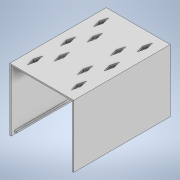
# Autodesk Inventor part: netzteil_halter_oben
Saved by Autodesk Inventor 2021 (Build 250183000, 183)
## iProperties
Created: 2021-11-10
Part Number: netzteil_halter_oben
Material: Generisch
Document SubType Name: Modeling
Designer: Simon
Density: 1 g/cm^3
Appearance: Vorgabe
Author: Simon
Autodesk Inventor part; units mm, degrees
ref_plane "YZ Plane" through (0, 0, 0) normal (1, 0, 0) x (0, 1, 0)
ref_plane "XZ Plane" through (0, 0, 0) normal (0, 1, 0) x (-1, 0, 0)
ref_plane "XY Plane" through (0, 0, 0) normal (0, 0, 1) x (1, 0, 0)
sketch "Skizze1" plane through (0, 0, 0) normal (0, 0, 1) x (1, 0, 0)
  line L0 (-63, 61.5) -> (63, 61.5)
  line L1 (63, 61.5) -> (63, -61.5)
  line L2 (63, -61.5) -> (-63, -61.5)
  line L3 (-63, -61.5) -> (-63, 61.5)
  point P0 (0, 0)
  point P1 (0, 61.5)
  point P2 (-63, 0)
  dimension "d0" = 123
  dimension "d1" = 126
  constraints: 8 end point, 2 midpoint, 2 parallel, 1 horizontal, 1 horizontal alignment, 1 perpendicular, 1 vertical alignment
  measures "d0" distance of L0.end L1.end
  measures "d1" distance between parallel lines of L1 L3
extrude "Extrusion1" add sketch "Skizze1" along normal blind 5
sketch "Skizze3" plane through (0, 0, 5) normal (0, 0, 1) x (1, 0, 0)
  line L0 (5, -51.5) -> (5, 58.5) construction
  line L1 (5, 58.5) -> (10.5, 58.5) construction
  line L2 (10.5, 58.5) -> (10.5, -51.5) construction
  line L3 (10.5, -51.5) -> (60, -51.5) construction
  line L4 (60, -51.5) -> (60, -54.5) construction
  line L5 (60, -54.5) -> (56, -54.5) construction
  line L6 (56, -54.5) -> (56, -58.5) construction
  line L7 (56, -58.5) -> (60, -58.5) construction
  line L8 (60, -58.5) -> (60, -61.5) construction
  line L9 (60, -61.5) -> (-60, -61.5) construction
  line L10 (-60, -61.5) -> (-60, -58.5) construction
  line L11 (-60, -58.5) -> (-56, -58.5) construction
  line L12 (-56, -58.5) -> (-56, -54.5) construction
  line L13 (-56, -54.5) -> (-60, -54.5) construction
  line L14 (-60, -54.5) -> (-60, -51.5) construction
  line L15 (-60, -51.5) -> (5, -51.5) construction
  line L16 (-63, -61.5) -> (63, -61.5) projected
  line L17 (63, -61.5) -> (63, 61.5) projected
  line L18 (-63, -61.5) -> (-60.5, -61.5)
  line L19 (-60.5, -58) -> (-60.5, -61.5)
  line L20 (-60.5, -58) -> (-56.5, -58)
  line L21 (-56.5, -58) -> (-56.5, -55)
  line L22 (-56.5, -55) -> (-60.5, -55)
  line L23 (-60.5, -55) -> (-60.5, 56.5)
  line L24 (60.5, 56.5) -> (60.5, -55)
  line L25 (60.5, -55) -> (56.5, -55)
  line L26 (56.5, -55) -> (56.5, -58)
  line L27 (56.5, -58) -> (60.5, -58)
  line L28 (60.5, -61.5) -> (60.5, -58)
  line L29 (60.5, -61.5) -> (63, -61.5)
  line L30 (63, -61.5) -> (63, 61.5)
  line L31 (63, 61.5) -> (-63, 61.5) projected
  line L32 (63, 61.5) -> (-63, 61.5)
  line L33 (-63, 61.5) -> (-63, -61.5)
  line L34 (4, 56.5) -> (4, 59)
  line L35 (4, 59) -> (11.5, 59)
  line L36 (11.5, 59) -> (11.5, 56.5)
  line L37 (-60.5, 56.5) -> (4, 56.5)
  line L38 (11.5, 56.5) -> (60.5, 56.5)
  point P0 (0, 0)
  dimension "d4" = 4
  dimension "d5" = 4
  dimension "d6" = 3
  dimension "d7" = 10
  dimension "d8" = 120
  dimension "d10" = 5.5
  dimension "d11" = 120
  dimension "d13" = 0.5
  dimension "d14" = 0.5
  dimension "d15" = 0.5
  dimension "d16" = 0.5
  dimension "d17" = 0.5
  dimension "d18" = 0.5
  dimension "d19" = 0.5
  dimension "d20" = 1
  dimension "d21" = 1
  dimension "d22" = 5
  dimension "d25" = 65
  constraints: 72 end point, 30 perpendicular, 15 point on line, 4 equal length, 2 collinear, 2 horizontal, 1 vertical
  measures "d4" distance of L10.end L11.end
  measures "d5" distance of L11.end L12.end
  measures "d6" distance between parallel lines of L9 L11
  measures "d7" distance between parallel lines of L15 L9
  measures "d8" distance of L8.end L9.end
  measures "d10" distance between parallel lines of L0 L2
  measures "d11" distance between parallel lines of L1 L9
  measures "d13" distance between parallel lines of L10 L19
  measures "d14" distance between parallel lines of L20 L11
  measures "d15" distance between parallel lines of L12 L21
  measures "d16" distance between parallel lines of L13 L22
  measures "d17" distance between parallel lines of L6 L26
  measures "d18" distance between parallel lines of L8 L28
  measures "d19" distance between parallel lines of L1 L35
  measures "d20" distance between parallel lines of L34 L0
  measures "d21" distance between parallel lines of L2 L36
  measures "d22" distance between parallel lines of L32 L38
  measures "d25" distance between parallel lines of L14 L0
extrude "Extrusion2" add sketch "Skizze3" along normal blind 179 contours L33 L31 L17 L16 L28 L27 L26 L25 L24 L38 L36 L35 L34 L37 L23 L22 L21 L20 L19
sketch "Skizze4" plane through (0, 0, 184) normal (0, 0, 1) x (1, 0, 0)
  line L0 (-63, -61.5) -> (63, -61.5) projected
  line L1 (63, 61.5) -> (-63, 61.5) projected
  line L2 (-63, -61.5) -> (-63, 61.5)
  line L3 (-63, 61.5) -> (63, 61.5)
  line L4 (63, 61.5) -> (63, -61.5)
  line L5 (-60.5, -61.5) -> (60.5, -61.5) projected
  line L6 (-63, -61.5) -> (-60.5, -61.5)
  line L7 (-60.5, -61.5) -> (-60.5, 59)
  line L8 (-60.5, 59) -> (60.5, 59)
  line L9 (60.5, 59) -> (60.5, -61.5)
  line L10 (60.5, -61.5) -> (63, -61.5)
  point P0 (0, 0)
  dimension "d26" = 2.5
  constraints: 16 end point, 6 perpendicular, 1 collinear, 1 vertical
  measures "d26" distance between parallel lines of L1 L8
extrude "Extrusion3" add sketch "Skizze4" along normal blind 6 contours L2 L1 L4 L0 L9 L8 L7
sketch "Skizze5" plane through (0, 0, 5) normal (0, 0, 1) x (1, 0, 0)
  line L0 (-60.5, -61.5) -> (60.5, -61.5) projected
  line L1 (-20, -61.5) -> (-20, -41.5)
  arc A0 (20, -41.5) -> (-20, -41.5) centre (0, -41.5) ccw
  line L2 (20, -41.5) -> (20, -61.5)
  line L3 (20, -61.5) -> (-20, -61.5)
  point P0 (0, 0)
  dimension "d29" = 40
  dimension "d30" = 20
  constraints: 6 end point, 2 point on circle, 2 point on line, 2 tangent, 1 centre point, 1 parallel, 1 perpendicular, 1 vertical, 1 vertical alignment
  measures "d29" distance between parallel lines of L1 L2
  measures "d30" distance from line of L0 A0.centre
extrude "Extrusion4" cut sketch "Skizze5" against normal up to surface (5 mm away)
sketch "Skizze6" plane through (-63, 61.5, 0) normal (0, 1, 0) x (1, 0, 0)
  line L0 (20, -15) -> (15.9808, -30)
  line L1 (15.9808, -30) -> (20, -45)
  line L2 (20, -45) -> (24.0192, -30)
  line L3 (24.0192, -30) -> (20, -15)
  line L4 (15.9808, -30) -> (24.0464, -30) construction
  line L5 (20, -15) -> (20, -45) construction
  line L6 (0, 0) -> (0, -190) projected
  line L7 (126, 0) -> (0, 0) projected
  line L8 (126, 0) -> (126, -190) projected
  point P0 (63, 0)
  point P1 (20, -30)
  point P2 (40, -62.5)
  point P3 (20, -95)
  point P4 (40, -127.5)
  point P5 (20, -160)
  point P6 (106, -160)
  point P7 (86, -127.5)
  point P8 (106, -95)
  point P9 (86, -62.5)
  point P10 (106, -30)
  point P11 (20.0136, -30)
  dimension "d33" = 30
  dimension "d34" = 30
  dimension "d37" = 20
  dimension "d38" = 30
  dimension "d39" = 65
  dimension "d40" = 65
  dimension "d41" = 20
  dimension "d42" = 32.5
  dimension "d43" = 65
  dimension "d44" = 20
  dimension "d45" = 20
  dimension "d46" = 190
  constraints: 12 end point, 7 vertical alignment, 5 horizontal alignment, 3 equal length, 2 midpoint, 1 horizontal, 1 vertical
  measures "d33" angle of L2 L1
  measures "d34" distance of L0.start L1.end
  measures "d37" distance from line of L6 point (20, -30)
  measures "d38" distance from line of L7 point (20, -30)
  measures "d39" distance of point (20, -95) point (20, -30)
  measures "d40" distance of point (20, -160) point (20, -95)
  measures "d41" horizontal distance of point (40, -62.5) point (20, -30)
  measures "d42" vertical distance of point (20, -30) point (40, -62.5)
  measures "d43" distance of point (40, -62.5) point (40, -127.5)
  measures "d44" distance from line of L8 point (106, -30)
  measures "d45" horizontal distance of point (106, -30) point (86, -62.5)
  measures "d46" distance of L6.start L6.end
extrude "Extrusion5" cut sketch "Skizze6" against normal up to surface (5 mm away)
pattern_sketch "Skizzenbasierte Anordnung1" of "Extrusion5" from (-43, 61.5, 30) copies at (-23, 61.5, 62.5) at (-43, 61.5, 95) at (-23, 61.5, 127.5) at (-43, 61.5, 160) at (43, 61.5, 160) at (23, 61.5, 127.5) at (43, 61.5, 95) at (23, 61.5, 62.5) at (43, 61.5, 30)
fillet "Rundung1" radius 1.4 6 edges at (58.5, -58, 184) (56.5, -56.5, 184) (58.5, -55, 184) (-58.5, -58, 184) (-56.5, -56.5, 184) (-58.5, -55, 184)
equation "\"d39\" = -d38 + 0.5 * d46"
equation "\"d40\" = d39"
equation "\"d42\" = 0.5 * d39"
equation "\"d43\" = d39"
equation "\"d44\" = d37"
equation "\"d45\" = d41"
